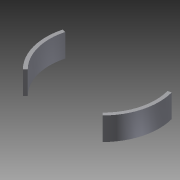
# Autodesk Inventor part: ss_inner_adapter
Saved by Autodesk Inventor 2011 SP2 (Build 150309200, 309)
## iProperties
Created: 2012-05-25
Part Number: ss_inner_adapter
Document SubType Name: Modeling
Designer: sungwook
Density: 1 g/cm^3
Author: sungwook
Autodesk Inventor part; units mm, degrees
ref_plane "YZ Plane" through (0, 0, 0) normal (1, 0, 0) x (0, 1, 0)
ref_plane "XZ Plane" through (0, 0, 0) normal (0, 1, 0) x (-1, 0, 0)
ref_plane "XY Plane" through (0, 0, 0) normal (0, 0, 1) x (1, 0, 0)
sketch "Sketch1" plane through (0, 0, 0) normal (0, 0, 1) x (1, 0, 0)
  circle A0 centre (0, 0) radius 12.25
  line L0 (-17.6349, 0) -> (17.6349, 0) projected
  line L1 (0, -17.15) -> (0, 17.15) projected
  line L2 (11.1081, 2.9764) -> (11.8326, 3.1705)
  line L3 (8.1317, -8.1317) -> (8.6621, -8.6621)
  line L4 (-11.1081, 2.9764) -> (-11.8326, 3.1705)
  line L5 (-8.1317, -8.1317) -> (-8.6621, -8.6621)
  arc A1 (-11.1081, 2.9764) -> (-8.1317, -8.1317) centre (0, 0) ccw
  arc A2 (8.1317, -8.1317) -> (11.1081, 2.9764) centre (0, 0) ccw
  dimension "d1" = 24.5
  dimension "d2" = 15
  dimension "d3" = 45
  constraints: 8 end point, 6 point on circle, 3 centre point, 2 coincident, 2 symmetric about line
  measures "d1" diameter of A0
  measures "d2" angle of L0 L2
  measures "d3" angle of L0 L3
extrude "Extrusion1" add sketch "Sketch1" along normal blind 5 contours L0 A2 L2 A0 | A0 L3 A2 L0
mirror "Mirror1" about plane through (0, 0, 0) normal (1, 0, 0) of "Extrusion1"
body "Solid1"
